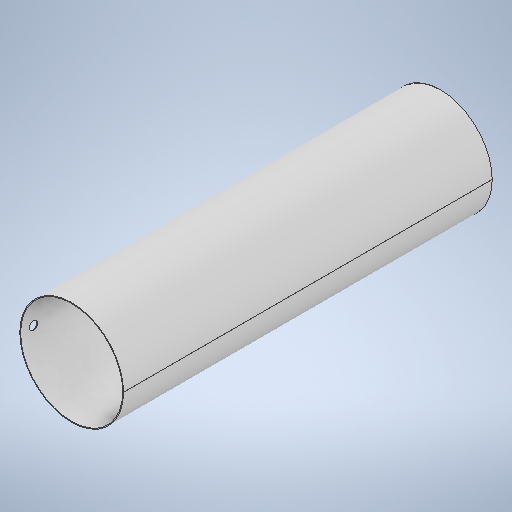
# Autodesk Inventor part: BSH 082 barrel wall
Saved by Autodesk Inventor 2025 (Build 290162010, 162A)
## iProperties
Created: 2024-08-04
Part Number: BSH 082 barrel wall
Material: Stainless Steel
Document SubType Name: Sheet Metal
Designer: pokla
Density: 8 g/cm^3
Sheet Metal Rule: AISI304 2mm Die16
Appearance: Default
Flat Pattern Width: 252.916 cm
Flat Pattern Length: 288.7 cm
Flat Pattern Area: 73016.8 cm^2
Sheet Metal Width: 2529,159 mm
Sheet Metal Length: 2887,000 mm
Sheet Metal Area: 7301682,012 mm^2
Author: pokla
Autodesk Inventor part; units mm, degrees
ref_plane "YZ Plane" through (0, 0, 0) normal (1, 0, 0) x (0, 1, 0)
ref_plane "XZ Plane" through (0, 0, 0) normal (0, 1, 0) x (-1, 0, 0)
ref_plane "XY Plane" through (0, 0, 0) normal (0, 0, 1) x (1, 0, 0)
sketch "Sketch1" plane through (0, 0, 0) normal (0, 0, 1) x (1, 0, 0)
  line L0 (406, 0) -> (400, 0)
  line L1 (400, 0) -> (400, 2887)
  line L2 (400, 2887) -> (406, 2887)
  line L3 (406, 2887) -> (406, 0)
  line L4 (0, 0) -> (0, 2896.1409)
  point P0 (403, 0)
  dimension "d0" = 6
  dimension "d1" = 2887
  dimension "d2" = 400
  constraints: 10 end point, 2 parallel, 2 perpendicular, 1 horizontal, 1 horizontal alignment, 1 midpoint
  measures "d0" distance of L1.end L2.end
  measures "d1" distance of L2.end L0.start
  measures "d2" distance of L4.start L0.end
revolve "Revolution1" add sketch "Sketch1" angle 359.9 about axis through (0, 0, 0) along (0, 1, 0)
sketch "Sketch2" plane through (0, 0, 0) normal (1, 0, 0) x (0, 1, 0)
  circle A0 centre (100, 0) radius 32.5
  point P0 (0, 0)
  dimension "d4" = 65
  dimension "d5" = 100
  constraints: 1 centre point
  measures "d4" diameter of A0
  measures "d5" distance of point (0, 0) A0.centre
extrude "Extrusion1" cut sketch "Sketch2" against normal through all
equation "\"BendReliefWidth\" = Thickness"
equation "\"BendReliefDepth\" = 0.5 * Thickness"
equation "\"CornerReliefSize\" = 4 * Thickness"
equation "\"MinimumRemnant\" = 2 * Thickness"
equation "\"TransitionRadius\" = BendRadius"
equation "\"JacobiRadiusSize\" = BendRadius"
equation "\"GapSize\" = Thickness"
equation "\"Thickness\" = 6"
equation "\"BendRadius\" = 2.75"
body "Solid1"
